Autodesk Inventor part; units mm, degrees
(part 7 of 11)
  arc A2531 (21.081, 10.0534) -> (21.1571, 10.058) centre (21.119, 10.0557) ccw
  line L1265 (21.082, 10.668) -> (21.119, 11.2803)
  arc A2532 (21.1571, 11.278) -> (21.081, 11.2826) centre (21.119, 11.2803) ccw
  arc A2533 (21.044, 10.6703) -> (21.12, 10.6657) centre (21.082, 10.668) ccw
  line L1266 (21.119, 11.2803) -> (21.2296, 11.8837)
  arc A2534 (21.2671, 11.8769) -> (21.1921, 11.8906) centre (21.2296, 11.8837) ccw
  arc A2535 (21.0816, 11.2872) -> (21.1565, 11.2735) centre (21.119, 11.2803) ccw
  line L1267 (21.2296, 11.8837) -> (21.4121, 12.4694)
  arc A2536 (21.4485, 12.4581) -> (21.3758, 12.4807) centre (21.4121, 12.4694) ccw
  arc A2537 (21.1933, 11.895) -> (21.266, 11.8724) centre (21.2296, 11.8837) ccw
  line L1268 (21.4121, 12.4694) -> (21.6639, 13.0288)
  arc A2538 (21.6986, 13.0132) -> (21.6291, 13.0444) centre (21.6639, 13.0288) ccw
  arc A2539 (21.3774, 12.485) -> (21.4469, 12.4537) centre (21.4121, 12.4694) ccw
  line L1269 (21.6639, 13.0288) -> (21.9812, 13.5538)
  arc A2540 (22.0138, 13.5341) -> (21.9486, 13.5735) centre (21.9812, 13.5538) ccw
  arc A2541 (21.6313, 13.0485) -> (21.6965, 13.0091) centre (21.6639, 13.0288) ccw
  line L1270 (21.9812, 13.5538) -> (22.3596, 14.0367)
  arc A2542 (22.3896, 14.0132) -> (22.3296, 14.0602) centre (22.3596, 14.0367) ccw
  arc A2543 (21.9512, 13.5773) -> (22.0112, 13.5303) centre (21.9812, 13.5538) ccw
  line L1271 (22.3596, 14.0367) -> (22.7933, 14.4704)
  arc A2544 (22.8203, 14.4435) -> (22.7664, 14.4974) centre (22.7933, 14.4704) ccw
  arc A2545 (22.3326, 14.0636) -> (22.3865, 14.0097) centre (22.3596, 14.0367) ccw
  line L1272 (22.7933, 14.4704) -> (23.2762, 14.8488)
  arc A2546 (23.2997, 14.8188) -> (23.2527, 14.8788) centre (23.2762, 14.8488) ccw
  arc A2547 (22.7698, 14.5004) -> (22.8168, 14.4404) centre (22.7933, 14.4704) ccw
  line L1273 (23.2762, 14.8488) -> (23.8012, 15.1661)
  arc A2548 (23.8209, 15.1335) -> (23.7815, 15.1987) centre (23.8012, 15.1661) ccw
  arc A2549 (23.2565, 14.8814) -> (23.2959, 14.8162) centre (23.2762, 14.8488) ccw
  line L1274 (23.8012, 15.1661) -> (24.3606, 15.4179)
  arc A2550 (24.3762, 15.3832) -> (24.3449, 15.4527) centre (24.3606, 15.4179) ccw
  arc A2551 (23.7855, 15.2009) -> (23.8168, 15.1314) centre (23.8012, 15.1661) ccw
  line L1275 (24.3606, 15.4179) -> (24.9463, 15.6003)
  arc A2552 (24.9576, 15.564) -> (24.9349, 15.6367) centre (24.9463, 15.6003) ccw
  arc A2553 (24.3492, 15.4543) -> (24.3719, 15.3815) centre (24.3606, 15.4179) ccw
  line L1276 (24.9463, 15.6003) -> (25.5497, 15.7109)
  arc A2554 (25.5566, 15.6734) -> (25.5428, 15.7483) centre (25.5497, 15.7108) ccw
  arc A2555 (24.9394, 15.6379) -> (24.9531, 15.5629) centre (24.9463, 15.6004) ccw
  line L1277 (25.5497, 15.7109) -> (26.162, 15.7478)
  arc A2556 (26.1643, 15.7098) -> (26.1597, 15.7858) centre (26.162, 15.7478) ccw
  arc A2557 (25.5474, 15.7489) -> (25.552, 15.6728) centre (25.5497, 15.7108) ccw
  line L1278 (26.162, 15.7478) -> (26.8194, 15.6894)
  arc A2558 (26.816, 15.6514) -> (26.8228, 15.7273) centre (26.8194, 15.6894) ccw
  arc A2559 (26.1654, 15.7858) -> (26.1586, 15.7099) centre (26.162, 15.7478) ccw
  line L1279 (26.8194, 15.6894) -> (27.464, 15.5482)
  arc A2560 (27.4559, 15.511) -> (27.4722, 15.5854) centre (27.464, 15.5482) ccw
  arc A2561 (26.8275, 15.7266) -> (26.8112, 15.6522) centre (26.8194, 15.6894) ccw
  line L1280 (27.464, 15.5482) -> (28.0857, 15.3267)
  arc A2562 (28.0729, 15.2908) -> (28.0985, 15.3626) centre (28.0857, 15.3267) ccw
  arc A2563 (27.4768, 15.5841) -> (27.4513, 15.5123) centre (27.464, 15.5482) ccw
  line L1281 (28.0857, 15.3267) -> (28.6745, 15.0285)
  arc A2564 (28.6573, 14.9945) -> (28.6917, 15.0625) centre (28.6745, 15.0285) ccw
  arc A2565 (28.1029, 15.3607) -> (28.0685, 15.2927) centre (28.0857, 15.3267) ccw
  line L1282 (28.6745, 15.0285) -> (29.2211, 14.6587)
  arc A2566 (29.1997, 14.6271) -> (29.2424, 14.6902) centre (29.2211, 14.6587) ccw
  arc A2567 (28.6959, 15.0601) -> (28.6532, 14.997) centre (28.6745, 15.0285) ccw
  line L1283 (29.2211, 14.6587) -> (29.7166, 14.2228)
  arc A2568 (29.691, 14.1936) -> (29.7413, 14.2507) centre (29.7162, 14.2222) ccw
  arc A2569 (29.2463, 14.6873) -> (29.1959, 14.6301) centre (29.2211, 14.6587) ccw
  line L1284 (29.7166, 14.2228) -> (29.8258, 13.5976)
  arc A2570 (29.7972, 13.5724) -> (29.8544, 13.6228) centre (29.8258, 13.5976) ccw
  arc A2571 (29.7447, 14.2473) -> (29.6876, 14.197) centre (29.7162, 14.2222) ccw
  line L1285 (29.8258, 13.5976) -> (29.8563, 12.9383)
  arc A2572 (30.491, 13.1592) -> (30.5541, 13.2019) centre (30.5225, 13.1805) ccw
  arc A2573 (29.8573, 13.6189) -> (29.7942, 13.5762) centre (29.8258, 13.5976) ccw
  line L1286 (29.8563, 12.9383) -> (29.8033, 12.2805)
  arc A2574 (29.7654, 12.2835) -> (29.8373, 12.2977) centre (29.8033, 12.2805) ccw
  arc A2575 (30.5565, 13.1977) -> (30.4885, 13.1633) centre (30.5225, 13.1805) ccw
  line L1287 (29.8033, 12.2805) -> (31.0422, 11.97)
  arc A2576 (31.0063, 11.9573) -> (31.0781, 11.9828) centre (31.0422, 11.97) ccw
  arc A2577 (29.8406, 12.2727) -> (29.7674, 12.2677) centre (29.8033, 12.2805) ccw
  line L1288 (31.0422, 11.97) -> (31.1834, 11.3254)
  arc A2578 (31.1462, 11.3172) -> (31.2206, 11.3335) centre (31.1834, 11.3254) ccw
  arc A2579 (31.0794, 11.9782) -> (31.005, 11.9619) centre (31.0422, 11.97) ccw
  line L1289 (31.1834, 11.3254) -> (31.3469, 10.7676)
  arc A2580 (31.3089, 10.7642) -> (31.3848, 10.771) centre (31.3469, 10.7676) ccw
  arc A2581 (31.2213, 11.3288) -> (31.1454, 11.322) centre (31.1834, 11.3254) ccw
  line L1290 (31.3469, 10.7676) -> (30.0789, 10.6966)
  arc A2582 (30.0753, 10.7345) -> (30.0789, 10.6585) centre (30.0789, 10.6966) ccw
  arc A2583 (31.3469, 10.7295) -> (31.3469, 10.8057) centre (31.3469, 10.7676) ccw
  line L1291 (30.0789, 10.6966) -> (30.0301, 11.2202)
  arc A2584 (30.0681, 11.2237) -> (29.9922, 11.2166) centre (30.0301, 11.2201) ccw
  arc A2585 (30.0408, 10.6952) -> (30.1169, 10.698) centre (30.0789, 10.6966) ccw
  line L1292 (30.0301, 11.2202) -> (29.9074, 11.7314)
  arc A2586 (29.9449, 11.7382) -> (29.8699, 11.7246) centre (29.9074, 11.7314) ccw
  arc A2587 (29.9926, 11.2133) -> (30.0676, 11.227) centre (30.0301, 11.2201) ccw
  line L1293 (29.9074, 11.7314) -> (29.7131, 12.22)
  arc A2588 (29.7281, 12.2215) -> (29.6558, 12.1974) centre (29.6919, 12.2094) ccw
  arc A2589 (29.8712, 11.7193) -> (29.9435, 11.7435) centre (29.9074, 11.7314) ccw
  line L1294 (29.7131, 12.22) -> (29.4514, 12.6758)
  arc A2590 (29.4855, 12.6929) -> (29.4174, 12.6587) centre (29.4514, 12.6758) ccw
  arc A2591 (29.6579, 12.1924) -> (29.726, 12.2265) centre (29.6919, 12.2094) ccw
  line L1295 (29.4514, 12.6758) -> (29.158, 13.1122)
  arc A2592 (29.1892, 13.134) -> (29.1267, 13.0905) centre (29.158, 13.1122) ccw
  arc A2593 (29.4201, 12.654) -> (29.4827, 12.6976) centre (29.4514, 12.6758) ccw
  line L1296 (29.158, 13.1122) -> (28.7968, 13.4952)
  arc A2594 (28.8247, 13.5212) -> (28.769, 13.4693) centre (28.7968, 13.4952) ccw
  arc A2595 (29.1301, 13.0862) -> (29.1858, 13.1382) centre (29.158, 13.1122) ccw
  line L1297 (28.7968, 13.4952) -> (28.387, 13.8247)
  arc A2596 (28.4109, 13.8544) -> (28.3631, 13.795) centre (28.387, 13.8247) ccw
  arc A2597 (28.773, 13.4655) -> (28.8207, 13.5249) centre (28.7968, 13.4952) ccw
  line L1298 (28.387, 13.8247) -> (27.9346, 14.0922)
  arc A2598 (27.9539, 14.125) -> (27.9152, 14.0595) centre (27.9345, 14.0923) ccw
  arc A2599 (28.3676, 13.7919) -> (28.4064, 13.8575) centre (28.387, 13.8247) ccw
  line L1299 (27.9346, 14.0922) -> (27.4486, 14.2929)
  arc A2600 (27.463, 14.3282) -> (27.4339, 14.2578) centre (27.4485, 14.293) ccw
  arc A2601 (27.92, 14.057) -> (27.9491, 14.1275) centre (27.9345, 14.0923) ccw
  line L1300 (27.4486, 14.2929) -> (26.939, 14.4224)
  arc A2602 (26.9482, 14.4594) -> (26.9295, 14.3855) centre (26.9388, 14.4224) ccw
  arc A2603 (27.4393, 14.256) -> (27.458, 14.3298) centre (27.4486, 14.2929) ccw
  line L1301 (26.939, 14.4224) -> (26.416, 14.478)
  arc A2604 (26.42, 14.5159) -> (26.412, 14.4401) centre (26.416, 14.478) ccw
  arc A2605 (26.9348, 14.3846) -> (26.9429, 14.4603) centre (26.9388, 14.4224) ccw
  line L1302 (26.416, 14.478) -> (26.162, 14.478)
  arc A2606 (26.162, 14.5161) -> (26.162, 14.4399) centre (26.162, 14.478) ccw
  arc A2607 (26.416, 14.4399) -> (26.416, 14.5161) centre (26.416, 14.478) ccw
  line L1303 (26.162, 14.478) -> (25.6198, 14.4392)
  arc A2608 (25.6171, 14.4772) -> (25.6225, 14.4012) centre (25.6198, 14.4392) ccw
  arc A2609 (26.1647, 14.44) -> (26.1593, 14.516) centre (26.162, 14.478) ccw
  line L1304 (25.6198, 14.4392) -> (25.0886, 14.3237)
  arc A2610 (25.0805, 14.3609) -> (25.0967, 14.2864) centre (25.0886, 14.3237) ccw
  arc A2611 (25.6279, 14.402) -> (25.6117, 14.4764) centre (25.6198, 14.4392) ccw
  line L1305 (25.0886, 14.3237) -> (24.5793, 14.1337)
  arc A2612 (24.566, 14.1694) -> (24.5926, 14.098) centre (24.5793, 14.1337) ccw
  arc A2613 (25.1019, 14.288) -> (25.0753, 14.3594) centre (25.0886, 14.3237) ccw
  line L1306 (24.5793, 14.1337) -> (24.1022, 13.8732)
  arc A2614 (24.0839, 13.9066) -> (24.1204, 13.8397) centre (24.1022, 13.8732) ccw
  arc A2615 (24.5975, 14.1003) -> (24.561, 14.1671) centre (24.5793, 14.1337) ccw
  line L1307 (24.1022, 13.8732) -> (23.667, 13.5474)
  arc A2616 (23.6441, 13.5779) -> (23.6898, 13.5169) centre (23.667, 13.5474) ccw
  arc A2617 (24.125, 13.8427) -> (24.0793, 13.9037) centre (24.1022, 13.8732) ccw
  line L1308 (23.667, 13.5474) -> (23.2826, 13.163)
  arc A2618 (23.2557, 13.19) -> (23.3095, 13.1361) centre (23.2826, 13.163) ccw
  arc A2619 (23.6939, 13.5205) -> (23.64, 13.5743) centre (23.667, 13.5474) ccw
  line L1309 (23.2826, 13.163) -> (22.9568, 12.7278)
  arc A2620 (22.9263, 12.7507) -> (22.9873, 12.705) centre (22.9568, 12.7278) ccw
  arc A2621 (23.3131, 13.1402) -> (23.2521, 13.1859) centre (23.2826, 13.163) ccw
  line L1310 (22.9568, 12.7278) -> (22.6963, 12.2507)
  arc A2622 (22.6629, 12.269) -> (22.7297, 12.2325) centre (22.6963, 12.2507) ccw
  arc A2623 (22.9903, 12.7096) -> (22.9234, 12.7461) centre (22.9568, 12.7278) ccw
  line L1311 (22.6963, 12.2507) -> (22.5063, 11.7414)
  arc A2624 (22.4706, 11.7547) -> (22.542, 11.7281) centre (22.5063, 11.7414) ccw
  arc A2625 (22.732, 12.2374) -> (22.6606, 12.264) centre (22.6963, 12.2507) ccw
  line L1312 (22.5063, 11.7414) -> (22.3908, 11.2102)
  arc A2626 (22.3535, 11.2183) -> (22.428, 11.2021) centre (22.3908, 11.2102) ccw
  arc A2627 (22.5436, 11.7333) -> (22.4691, 11.7495) centre (22.5063, 11.7414) ccw
  line L1313 (22.3908, 11.2102) -> (22.352, 10.668)
  arc A2628 (22.314, 10.6707) -> (22.39, 10.6653) centre (22.352, 10.668) ccw
  arc A2629 (22.4288, 11.2075) -> (22.3528, 11.2129) centre (22.3908, 11.2102) ccw
  line L1314 (22.352, 10.668) -> (22.3908, 10.1258)
  arc A2630 (22.3528, 10.1231) -> (22.4288, 10.1285) centre (22.3908, 10.1258) ccw
  arc A2631 (22.39, 10.6707) -> (22.314, 10.6653) centre (22.352, 10.668) ccw
  line L1315 (22.3908, 10.1258) -> (22.5063, 9.5946)
  arc A2632 (22.4691, 9.5865) -> (22.5436, 9.6027) centre (22.5063, 9.5946) ccw
  arc A2633 (22.428, 10.1339) -> (22.3535, 10.1177) centre (22.3908, 10.1258) ccw
  line L1316 (22.5063, 9.5946) -> (22.6963, 9.0853)
  arc A2634 (22.6606, 9.072) -> (22.732, 9.0986) centre (22.6963, 9.0853) ccw
  arc A2635 (22.542, 9.6079) -> (22.4706, 9.5813) centre (22.5063, 9.5946) ccw
  line L1317 (22.6963, 9.0853) -> (22.9568, 8.6082)
  arc A2636 (22.9234, 8.5899) -> (22.9903, 8.6264) centre (22.9568, 8.6082) ccw
  arc A2637 (22.7297, 9.1035) -> (22.6629, 9.067) centre (22.6963, 9.0853) ccw
  line L1318 (22.9568, 8.6082) -> (23.2826, 8.173)
  arc A2638 (23.2521, 8.1501) -> (23.3131, 8.1958) centre (23.2826, 8.173) ccw
  arc A2639 (22.9873, 8.631) -> (22.9263, 8.5853) centre (22.9568, 8.6082) ccw
  line L1319 (23.2826, 8.173) -> (23.667, 7.7886)
  arc A2640 (23.64, 7.7617) -> (23.6939, 7.8155) centre (23.667, 7.7886) ccw
  arc A2641 (23.3095, 8.1999) -> (23.2557, 8.146) centre (23.2826, 8.173) ccw
  line L1320 (23.667, 7.7886) -> (24.1022, 7.4628)
  arc A2642 (24.0793, 7.4323) -> (24.125, 7.4933) centre (24.1022, 7.4628) ccw
  arc A2643 (23.6898, 7.8191) -> (23.6441, 7.7581) centre (23.667, 7.7886) ccw
  line L1321 (24.1022, 7.4628) -> (24.5793, 7.2023)
  arc A2644 (24.561, 7.1689) -> (24.5975, 7.2357) centre (24.5793, 7.2023) ccw
  arc A2645 (24.1204, 7.4963) -> (24.0839, 7.4294) centre (24.1022, 7.4628) ccw
  line L1322 (24.5793, 7.2023) -> (25.0886, 7.0123)
  arc A2646 (25.0753, 6.9766) -> (25.1019, 7.048) centre (25.0886, 7.0123) ccw
  arc A2647 (24.5926, 7.238) -> (24.566, 7.1666) centre (24.5793, 7.2023) ccw
  line L1323 (25.0886, 7.0123) -> (25.6198, 6.8968)
  arc A2648 (25.6117, 6.8595) -> (25.6279, 6.934) centre (25.6198, 6.8968) ccw
  arc A2649 (25.0967, 7.0496) -> (25.0805, 6.9751) centre (25.0886, 7.0123) ccw
  line L1324 (25.6198, 6.8968) -> (26.162, 6.858)
  arc A2650 (26.1593, 6.82) -> (26.1647, 6.896) centre (26.162, 6.858) ccw
  arc A2651 (25.6225, 6.9348) -> (25.6171, 6.8588) centre (25.6198, 6.8968) ccw
  line L1325 (26.162, 6.858) -> (26.6485, 6.8782)
  arc A2652 (26.65, 6.8402) -> (26.6469, 6.9163) centre (26.6485, 6.8782) ccw
  arc A2653 (26.1604, 6.8961) -> (26.1636, 6.8199) centre (26.162, 6.858) ccw
  line L1326 (26.6485, 6.8782) -> (27.1281, 6.9618)
  arc A2654 (27.1347, 6.9242) -> (27.1216, 6.9993) centre (27.1281, 6.9618) ccw
  arc A2655 (26.6419, 6.9158) -> (26.655, 6.8407) centre (26.6485, 6.8782) ccw
  line L1327 (27.1281, 6.9618) -> (27.5928, 7.1072)
  arc A2656 (27.6042, 7.0709) -> (27.5814, 7.1436) centre (27.5928, 7.1072) ccw
  arc A2657 (27.1167, 6.9982) -> (27.1395, 6.9254) centre (27.1281, 6.9618) ccw
  line L1328 (27.5928, 7.1072) -> (28.0345, 7.3121)
  arc A2658 (28.0505, 7.2775) -> (28.0184, 7.3466) centre (28.0345, 7.3121) ccw
  arc A2659 (27.5767, 7.1418) -> (27.6088, 7.0726) centre (27.5928, 7.1072) ccw
  line L1329 (28.0345, 7.3121) -> (28.4456, 7.5728)
  arc A2660 (28.466, 7.5406) -> (28.4252, 7.605) centre (28.4456, 7.5728) ccw
  arc A2661 (28.0141, 7.3443) -> (28.0549, 7.2799) centre (28.0345, 7.3121) ccw
  line L1330 (28.4456, 7.5728) -> (28.8192, 7.885)
  arc A2662 (28.8437, 7.8558) -> (28.7948, 7.9143) centre (28.8192, 7.885) ccw
  arc A2663 (28.4212, 7.602) -> (28.4701, 7.5436) centre (28.4456, 7.5728) ccw
  line L1331 (28.8192, 7.885) -> (29.1489, 8.2433)
  arc A2664 (29.177, 8.2175) -> (29.1209, 8.2691) centre (29.1489, 8.2433) ccw
  arc A2665 (28.7912, 7.9108) -> (28.8473, 7.8592) centre (28.8192, 7.885) ccw
  line L1332 (29.1489, 8.2433) -> (29.429, 8.6416)
  arc A2666 (29.4602, 8.6196) -> (29.3979, 8.6635) centre (29.429, 8.6416) ccw
  arc A2667 (29.1178, 8.2652) -> (29.1801, 8.2214) centre (29.1489, 8.2433) ccw
  line L1333 (29.429, 8.6416) -> (29.6547, 9.073)
  arc A2668 (29.6885, 9.0553) -> (29.621, 9.0906) centre (29.6547, 9.073) ccw
  arc A2669 (29.3953, 8.6592) -> (29.4628, 8.6239) centre (29.429, 8.6416) ccw
  line L1334 (29.6547, 9.073) -> (29.2095, 9.27)
  arc A2670 (29.858, 9.517) -> (29.7864, 9.5432) centre (29.8222, 9.5301) ccw
  arc A2671 (29.619, 9.0861) -> (29.6905, 9.0598) centre (29.6547, 9.073) ccw
  line L1335 (29.2095, 9.27) -> (28.7423, 9.4072)
  arc A2672 (28.7795, 9.3988) -> (28.7051, 9.4155) centre (28.7423, 9.4072) ccw
  arc A2673 (29.1723, 9.2783) -> (29.2467, 9.2616) centre (29.2095, 9.27) ccw
  line L1336 (28.7423, 9.4072) -> (28.2613, 9.4822)
  arc A2674 (28.2992, 9.4788) -> (28.2233, 9.4856) centre (28.2613, 9.4822) ccw
  arc A2675 (28.7044, 9.4106) -> (28.7803, 9.4038) centre (28.7423, 9.4072) ccw
  line L1337 (28.2613, 9.4822) -> (28.3443, 10.7495)
  arc A2676 (28.3443, 10.7114) -> (28.3443, 10.7876) centre (28.3443, 10.7495) ccw
  arc A2677 (28.2613, 9.5203) -> (28.2846, 9.4521) centre (28.2613, 9.4822) ccw
  line L1338 (21.1328, 9.9806) -> (21.1328, 11.3554)
  arc A2678 (21.1709, 11.3554) -> (21.0947, 11.3554) centre (21.1328, 11.3554) ccw
  arc A2679 (21.0947, 9.9806) -> (21.1709, 9.9806) centre (21.1328, 9.9806) ccw
  line L1339 (21.2852, 9.2739) -> (21.2852, 12.0621)
  arc A2680 (21.3233, 12.0621) -> (21.2471, 12.0621) centre (21.2852, 12.0621) ccw
  arc A2681 (21.2471, 9.2739) -> (21.3233, 9.2739) centre (21.2852, 9.2739) ccw
  line L1340 (21.4376, 8.81) -> (21.4376, 12.526)
  arc A2682 (21.4757, 12.526) -> (21.3995, 12.526) centre (21.4376, 12.526) ccw
  arc A2683 (21.3995, 8.81) -> (21.4757, 8.81) centre (21.4376, 8.81) ccw
  line L1341 (21.59, 8.4714) -> (21.59, 12.8646)
  arc A2684 (21.6281, 12.8646) -> (21.5519, 12.8646) centre (21.59, 12.8646) ccw
  arc A2685 (21.5519, 8.4714) -> (21.6281, 8.4714) centre (21.59, 8.4714) ccw
  line L1342 (21.7424, 8.1773) -> (21.7424, 13.1587)
  arc A2686 (21.7805, 13.1587) -> (21.7043, 13.1587) centre (21.7424, 13.1587) ccw
  arc A2687 (21.7043, 8.1773) -> (21.7805, 8.1773) centre (21.7424, 8.1773) ccw
  line L1343 (21.8948, 7.9252) -> (21.8948, 13.4108)
  arc A2688 (21.9329, 13.4108) -> (21.8567, 13.4108) centre (21.8948, 13.4108) ccw
  arc A2689 (21.8567, 7.9252) -> (21.9329, 7.9252) centre (21.8948, 7.9252) ccw
  line L1344 (22.0472, 7.698) -> (22.0472, 13.6379)
  arc A2690 (22.0853, 13.6379) -> (22.0091, 13.6379) centre (22.0472, 13.6379) ccw
  arc A2691 (22.0091, 7.698) -> (22.0853, 7.698) centre (22.0472, 7.698) ccw
  line L1345 (22.1996, 7.5035) -> (22.1996, 13.8325)
  arc A2692 (22.2377, 13.8325) -> (22.1615, 13.8325) centre (22.1996, 13.8325) ccw
  arc A2693 (22.1615, 7.5035) -> (22.2377, 7.5035) centre (22.1996, 7.5035) ccw
  line L1346 (22.352, 7.309) -> (22.352, 10.668)
  arc A2694 (22.3901, 10.668) -> (22.3139, 10.668) centre (22.352, 10.668) ccw
  arc A2695 (22.3139, 7.309) -> (22.3901, 7.309) centre (22.352, 7.309) ccw
  line L1347 (22.352, 10.668) -> (22.352, 14.027)
  arc A2696 (22.3901, 14.027) -> (22.3139, 14.027) centre (22.352, 14.027) ccw
  arc A2697 (22.3139, 10.668) -> (22.3901, 10.668) centre (22.352, 10.668) ccw
  line L1348 (22.5044, 7.1545) -> (22.5044, 9.6035)
  arc A2698 (22.5425, 9.6035) -> (22.4663, 9.6035) centre (22.5044, 9.6035) ccw
  arc A2699 (22.4663, 7.1545) -> (22.5425, 7.1545) centre (22.5044, 7.1545) ccw
  line L1349 (22.5044, 11.7325) -> (22.5044, 14.1815)
  arc A2700 (22.5425, 14.1815) -> (22.4663, 14.1815) centre (22.5044, 14.1815) ccw
  arc A2701 (22.4663, 11.7325) -> (22.5425, 11.7325) centre (22.5044, 11.7325) ccw
  line L1350 (22.6568, 7.0021) -> (22.6568, 9.1912)
  arc A2702 (22.6949, 9.1912) -> (22.6187, 9.1912) centre (22.6568, 9.1912) ccw
  arc A2703 (22.6187, 7.0021) -> (22.6949, 7.0021) centre (22.6568, 7.0021) ccw
  line L1351 (22.6568, 12.1448) -> (22.6568, 14.3339)
  arc A2704 (22.6949, 14.3339) -> (22.6187, 14.3339) centre (22.6568, 14.3339) ccw
  arc A2705 (22.6187, 12.1448) -> (22.6949, 12.1448) centre (22.6568, 12.1448) ccw
  line L1352 (22.8092, 6.8531) -> (22.8092, 8.8785)
  arc A2706 (22.8473, 8.8785) -> (22.7711, 8.8785) centre (22.8092, 8.8785) ccw
  arc A2707 (22.7711, 6.8531) -> (22.8473, 6.8531) centre (22.8092, 6.8531) ccw
  line L1353 (22.8092, 12.4575) -> (22.8092, 14.4828)
  arc A2708 (22.8473, 14.4828) -> (22.7711, 14.4828) centre (22.8092, 14.4828) ccw
  arc A2709 (22.7711, 12.4575) -> (22.8473, 12.4575) centre (22.8092, 12.4575) ccw
  line L1354 (22.9616, 6.7337) -> (22.9616, 8.6018)
  arc A2710 (22.9997, 8.6018) -> (22.9235, 8.6018) centre (22.9616, 8.6018) ccw
  arc A2711 (22.9235, 6.7337) -> (22.9997, 6.7337) centre (22.9616, 6.7337) ccw
  line L1355 (22.9616, 12.7342) -> (22.9616, 14.6023)
  arc A2712 (22.9997, 14.6023) -> (22.9235, 14.6023) centre (22.9616, 14.6023) ccw
  arc A2713 (22.9235, 12.7342) -> (22.9997, 12.7342) centre (22.9616, 12.7342) ccw
  line L1356 (23.114, 6.6143) -> (23.114, 8.3982)
  arc A2714 (23.1521, 8.3982) -> (23.0759, 8.3982) centre (23.114, 8.3982) ccw
  arc A2715 (23.0759, 6.6143) -> (23.1521, 6.6143) centre (23.114, 6.6143) ccw
  line L1357 (23.114, 12.9378) -> (23.114, 14.7217)
  arc A2716 (23.1521, 14.7217) -> (23.0759, 14.7217) centre (23.114, 14.7217) ccw
  arc A2717 (23.0759, 12.9378) -> (23.1521, 12.9378) centre (23.114, 12.9378) ccw
  line L1358 (23.2664, 6.4949) -> (23.2664, 8.1946)
  arc A2718 (23.3045, 8.1946) -> (23.2283, 8.1946) centre (23.2664, 8.1946) ccw
  arc A2719 (23.2283, 6.4949) -> (23.3045, 6.4949) centre (23.2664, 6.4949) ccw
  line L1359 (23.2664, 13.1414) -> (23.2664, 14.8411)
  arc A2720 (23.3045, 14.8411) -> (23.2283, 14.8411) centre (23.2664, 14.8411) ccw
  arc A2721 (23.2283, 13.1414) -> (23.3045, 13.1414) centre (23.2664, 13.1414) ccw
  line L1360 (23.4187, 6.401) -> (23.4188, 8.0367)
  arc A2722 (23.4569, 8.0367) -> (23.3807, 8.0367) centre (23.4188, 8.0367) ccw
  arc A2723 (23.3806, 6.401) -> (23.4568, 6.401) centre (23.4187, 6.401) ccw
  line L1361 (23.4188, 13.2993) -> (23.4188, 14.935)
  arc A2724 (23.4569, 14.935) -> (23.3807, 14.935) centre (23.4188, 14.935) ccw
  arc A2725 (23.3807, 13.2993) -> (23.4569, 13.2993) centre (23.4188, 13.2993) ccw
  line L1362 (23.5711, 6.3089) -> (23.5712, 7.8843)
  arc A2726 (23.6093, 7.8843) -> (23.5331, 7.8843) centre (23.5712, 7.8843) ccw
  arc A2727 (23.533, 6.3089) -> (23.6092, 6.3089) centre (23.5711, 6.3089) ccw
  line L1363 (23.5712, 13.4517) -> (23.5712, 15.0271)
  arc A2728 (23.6093, 15.0271) -> (23.5331, 15.0271) centre (23.5712, 15.0271) ccw
  arc A2729 (23.5331, 13.4517) -> (23.6093, 13.4517) centre (23.5712, 13.4517) ccw
  line L1364 (23.7235, 6.2167) -> (23.7236, 7.7462)
  arc A2730 (23.7617, 7.7462) -> (23.6855, 7.7462) centre (23.7236, 7.7462) ccw
  arc A2731 (23.6854, 6.2167) -> (23.7616, 6.2167) centre (23.7235, 6.2167) ccw
  line L1365 (23.7236, 13.5898) -> (23.7236, 15.1192)
  arc A2732 (23.7617, 15.1192) -> (23.6855, 15.1192) centre (23.7236, 15.1192) ccw
  arc A2733 (23.6855, 13.5898) -> (23.7617, 13.5898) centre (23.7236, 13.5898) ccw
  line L1366 (23.8759, 6.1361) -> (23.876, 7.632)
  arc A2734 (23.9141, 7.632) -> (23.8379, 7.632) centre (23.876, 7.632) ccw
  arc A2735 (23.8378, 6.1361) -> (23.914, 6.1361) centre (23.8759, 6.1361) ccw
  line L1367 (23.876, 13.7039) -> (23.876, 15.1998)
  arc A2736 (23.9141, 15.1998) -> (23.8379, 15.1998) centre (23.876, 15.1998) ccw
  arc A2737 (23.8379, 13.7039) -> (23.9141, 13.7039) centre (23.876, 13.7039) ccw
  line L1368 (24.0283, 6.0675) -> (24.0284, 7.518)
  arc A2738 (24.0665, 7.518) -> (23.9903, 7.518) centre (24.0284, 7.518) ccw
  arc A2739 (23.9902, 6.0675) -> (24.0664, 6.0675) centre (24.0283, 6.0675) ccw
  line L1369 (24.0284, 13.8179) -> (24.0284, 15.2684)
  arc A2740 (24.0665, 15.2684) -> (23.9903, 15.2684) centre (24.0284, 15.2684) ccw
  arc A2741 (23.9903, 13.8179) -> (24.0665, 13.8179) centre (24.0284, 13.8179) ccw
  line L1370 (24.1807, 5.9989) -> (24.1808, 7.4199)
  arc A2742 (24.2189, 7.4199) -> (24.1427, 7.4199) centre (24.1808, 7.4199) ccw
  arc A2743 (24.1426, 5.9989) -> (24.2188, 5.9989) centre (24.1807, 5.9989) ccw
  line L1371 (24.1808, 13.9161) -> (24.1808, 15.337)
  arc A2744 (24.2189, 15.337) -> (24.1427, 15.337) centre (24.1808, 15.337) ccw
  arc A2745 (24.1427, 13.9161) -> (24.2189, 13.9161) centre (24.1808, 13.9161) ccw
  line L1372 (24.3332, 5.9304) -> (24.3332, 7.3367)
  arc A2746 (24.3713, 7.3367) -> (24.2951, 7.3367) centre (24.3332, 7.3367) ccw
  arc A2747 (24.2951, 5.9304) -> (24.3713, 5.9304) centre (24.3332, 5.9304) ccw
  line L1373 (24.3332, 13.9993) -> (24.3332, 15.4056)
  arc A2748 (24.3713, 15.4056) -> (24.2951, 15.4056) centre (24.3332, 15.4056) ccw
  arc A2749 (24.2951, 13.9993) -> (24.3713, 13.9993) centre (24.3332, 13.9993) ccw
  line L1374 (24.4856, 5.8792) -> (24.4856, 7.2534)
  arc A2750 (24.5237, 7.2534) -> (24.4475, 7.2534) centre (24.4856, 7.2534) ccw
  arc A2751 (24.4475, 5.8792) -> (24.5237, 5.8792) centre (24.4856, 5.8792) ccw
  line L1375 (24.4856, 14.0825) -> (24.4856, 15.4568)
  arc A2752 (24.5237, 15.4568) -> (24.4475, 15.4568) centre (24.4856, 15.4568) ccw
  arc A2753 (24.4475, 14.0825) -> (24.5237, 14.0825) centre (24.4856, 14.0825) ccw
  line L1376 (24.638, 5.8317) -> (24.638, 7.1804)
  arc A2754 (24.6761, 7.1804) -> (24.5999, 7.1804) centre (24.638, 7.1804) ccw
  arc A2755 (24.5999, 5.8317) -> (24.6761, 5.8317) centre (24.638, 5.8317) ccw
  line L1377 (24.638, 14.1556) -> (24.638, 15.5043)
  arc A2756 (24.6761, 15.5043) -> (24.5999, 15.5043) centre (24.638, 15.5043) ccw
  arc A2757 (24.5999, 14.1556) -> (24.6761, 14.1556) centre (24.638, 14.1556) ccw
  line L1378 (24.7904, 5.7843) -> (24.7904, 7.1235)
  arc A2758 (24.8285, 7.1235) -> (24.7523, 7.1235) centre (24.7904, 7.1235) ccw
  arc A2759 (24.7523, 5.7843) -> (24.8285, 5.7843) centre (24.7904, 5.7843) ccw
  line L1379 (24.7904, 14.2124) -> (24.7904, 15.5518)
  arc A2760 (24.8285, 15.5518) -> (24.7523, 15.5518) centre (24.7904, 15.5518) ccw
  arc A2761 (24.7523, 14.2124) -> (24.8285, 14.2124) centre (24.7904, 14.2124) ccw
  line L1380 (24.9428, 5.7367) -> (24.9428, 7.0667)
  arc A2762 (24.9809, 7.0667) -> (24.9047, 7.0667) centre (24.9428, 7.0667) ccw
  arc A2763 (24.9047, 5.7367) -> (24.9809, 5.7367) centre (24.9428, 5.7367) ccw
  line L1381 (24.9428, 14.2693) -> (24.9428, 15.5993)
  arc A2764 (24.9809, 15.5993) -> (24.9047, 15.5993) centre (24.9428, 15.5993) ccw
  arc A2765 (24.9047, 14.2693) -> (24.9809, 14.2693) centre (24.9428, 14.2693) ccw
  line L1382 (25.0952, 5.7083) -> (25.0952, 7.0109)
  arc A2766 (25.1333, 7.0109) -> (25.0571, 7.0109) centre (25.0952, 7.0109) ccw
  arc A2767 (25.0571, 5.7083) -> (25.1333, 5.7083) centre (25.0952, 5.7083) ccw
  line L1383 (25.0952, 14.3251) -> (25.0952, 15.6277)
  arc A2768 (25.1333, 15.6277) -> (25.0571, 15.6277) centre (25.0952, 15.6277) ccw
  arc A2769 (25.0571, 14.3251) -> (25.1333, 14.3251) centre (25.0952, 14.3251) ccw
  line L1384 (25.2476, 5.6807) -> (25.2476, 6.9777)
  arc A2770 (25.2857, 6.9777) -> (25.2095, 6.9777) centre (25.2476, 6.9777) ccw
  arc A2771 (25.2095, 5.6807) -> (25.2857, 5.6807) centre (25.2476, 5.6807) ccw
  line L1385 (25.2476, 14.3583) -> (25.2476, 15.6555)
  arc A2772 (25.2857, 15.6555) -> (25.2095, 15.6555) centre (25.2476, 15.6555) ccw
  arc A2773 (25.2095, 14.3583) -> (25.2857, 14.3583) centre (25.2476, 14.3583) ccw
  line L1386 (25.4, 5.6528) -> (25.4, 6.9446)
  arc A2774 (25.4381, 6.9446) -> (25.3619, 6.9446) centre (25.4, 6.9446) ccw
  arc A2775 (25.3619, 5.6528) -> (25.4381, 5.6528) centre (25.4, 5.6528) ccw
  line L1387 (25.4, 14.3914) -> (25.4, 15.6834)
  arc A2776 (25.4381, 15.6834) -> (25.3619, 15.6834) centre (25.4, 15.6834) ccw
  arc A2777 (25.3619, 14.3914) -> (25.4381, 14.3914) centre (25.4, 14.3914) ccw
  line L1388 (25.5524, 5.6249) -> (25.5524, 6.9114)
  arc A2778 (25.5905, 6.9114) -> (25.5143, 6.9114) centre (25.5524, 6.9114) ccw
  arc A2779 (25.5143, 5.6249) -> (25.5905, 5.6249) centre (25.5524, 5.6249) ccw
  line L1389 (25.5524, 14.4246) -> (25.5524, 15.7111)
  arc A2780 (25.5905, 15.7111) -> (25.5143, 15.7111) centre (25.5524, 15.7111) ccw
  arc A2781 (25.5143, 14.4246) -> (25.5905, 14.4246) centre (25.5524, 14.4246) ccw
  line L1390 (25.7049, 5.6161) -> (25.7043, 6.8912)
  arc A2782 (25.7424, 6.8912) -> (25.6662, 6.8912) centre (25.7043, 6.8912) ccw
  arc A2783 (25.6668, 5.6161) -> (25.743, 5.6161) centre (25.7049, 5.6161) ccw
  line L1391 (25.7047, 14.4452) -> (25.7048, 15.7202)
  arc A2784 (25.7429, 15.7202) -> (25.6667, 15.7202) centre (25.7048, 15.7202) ccw
  arc A2785 (25.6666, 14.4452) -> (25.7428, 14.4452) centre (25.7047, 14.4452) ccw
  line L1392 (25.8573, 5.607) -> (25.8572, 6.8798)
  arc A2786 (25.8953, 6.8798) -> (25.8191, 6.8798) centre (25.8572, 6.8798) ccw
  arc A2787 (25.8192, 5.607) -> (25.8954, 5.607) centre (25.8573, 5.607) ccw
  line L1393 (25.8572, 14.4562) -> (25.8572, 15.7294)
  arc A2788 (25.8953, 15.7294) -> (25.8191, 15.7294) centre (25.8572, 15.7294) ccw
  arc A2789 (25.8191, 14.4562) -> (25.8953, 14.4562) centre (25.8572, 14.4562) ccw
  line L1394 (26.0097, 5.5978) -> (26.0096, 6.8689)
  arc A2790 (26.0477, 6.8689) -> (25.9715, 6.8689) centre (26.0096, 6.8689) ccw
  arc A2791 (25.9716, 5.5978) -> (26.0478, 5.5978) centre (26.0097, 5.5978) ccw
  line L1395 (26.0096, 14.4671) -> (26.0096, 15.7386)
  arc A2792 (26.0477, 15.7386) -> (25.9715, 15.7386) centre (26.0096, 15.7386) ccw
  arc A2793 (25.9715, 14.4671) -> (26.0477, 14.4671) centre (26.0096, 14.4671) ccw
  line L1396 (26.1621, 5.5887) -> (26.162, 6.858)
  arc A2794 (26.2001, 6.858) -> (26.1239, 6.858) centre (26.162, 6.858) ccw
  arc A2795 (26.124, 5.5887) -> (26.2002, 5.5887) centre (26.1621, 5.5887) ccw
  line L1397 (26.162, 14.478) -> (26.162, 15.7478)
  arc A2796 (26.2001, 15.7478) -> (26.1239, 15.7478) centre (26.162, 15.7478) ccw
  arc A2797 (26.1239, 14.478) -> (26.2001, 14.478) centre (26.162, 14.478) ccw
  line L1398 (26.3144, 5.5953) -> (26.3144, 6.8643)
  arc A2798 (26.3525, 6.8643) -> (26.2763, 6.8643) centre (26.3144, 6.8643) ccw
  arc A2799 (26.2763, 5.5953) -> (26.3525, 5.5953) centre (26.3144, 5.5953) ccw
  line L1399 (26.3148, 14.478) -> (26.3144, 15.7343)
  arc A2800 (26.3525, 15.7343) -> (26.2763, 15.7343) centre (26.3144, 15.7343) ccw
  arc A2801 (26.2767, 14.478) -> (26.3529, 14.478) centre (26.3148, 14.478) ccw
  line L1400 (26.4669, 5.6019) -> (26.4668, 6.8707)
  arc A2802 (26.5049, 6.8707) -> (26.4287, 6.8707) centre (26.4668, 6.8707) ccw
  arc A2803 (26.4288, 5.6019) -> (26.505, 5.6019) centre (26.4669, 5.6019) ccw
  line L1401 (26.4672, 14.4725) -> (26.4668, 15.7207)
  arc A2804 (26.5049, 15.7207) -> (26.4287, 15.7207) centre (26.4668, 15.7207) ccw
  arc A2805 (26.4291, 14.4725) -> (26.5053, 14.4725) centre (26.4672, 14.4725) ccw
  line L1402 (26.6193, 5.6085) -> (26.6192, 6.877)
  arc A2806 (26.6573, 6.877) -> (26.5811, 6.877) centre (26.6192, 6.877) ccw
  arc A2807 (26.5812, 5.6085) -> (26.6574, 5.6085) centre (26.6193, 5.6085) ccw
  line L1403 (26.6196, 14.4563) -> (26.6192, 15.7072)
  arc A2808 (26.6573, 15.7072) -> (26.5811, 15.7072) centre (26.6192, 15.7072) ccw
  arc A2809 (26.5815, 14.4563) -> (26.6577, 14.4563) centre (26.6196, 14.4563) ccw
  line L1404 (26.7717, 5.615) -> (26.7716, 6.8997)
  arc A2810 (26.8097, 6.8997) -> (26.7335, 6.8997) centre (26.7716, 6.8997) ccw
  arc A2811 (26.7336, 5.615) -> (26.8098, 5.615) centre (26.7717, 5.615) ccw
  line L1405 (26.772, 14.4402) -> (26.7716, 15.6936)
  arc A2812 (26.8097, 15.6936) -> (26.7335, 15.6936) centre (26.7716, 15.6936) ccw
  arc A2813 (26.7339, 14.4402) -> (26.8101, 14.4402) centre (26.772, 14.4402) ccw
  line L1406 (26.924, 5.6389) -> (26.924, 6.9262)
  arc A2814 (26.9621, 6.9262) -> (26.8859, 6.9262) centre (26.924, 6.9262) ccw
  arc A2815 (26.8859, 5.6389) -> (26.9621, 5.6389) centre (26.924, 5.6389) ccw
  line L1407 (26.9242, 14.4239) -> (26.924, 15.6665)
  arc A2816 (26.9621, 15.6665) -> (26.8859, 15.6665) centre (26.924, 15.6665) ccw
  arc A2817 (26.8861, 14.4239) -> (26.9623, 14.4239) centre (26.9242, 14.4239) ccw
  line L1408 (27.0758, 5.6694) -> (27.0764, 6.9528)
  arc A2818 (27.1145, 6.9528) -> (27.0383, 6.9528) centre (27.0764, 6.9528) ccw
  arc A2819 (27.0377, 5.6694) -> (27.1139, 5.6694) centre (27.0758, 5.6694) ccw
  line L1409 (27.0764, 14.3875) -> (27.0764, 15.6331)
  arc A2820 (27.1145, 15.6331) -> (27.0383, 15.6331) centre (27.0764, 15.6331) ccw
  arc A2821 (27.0383, 14.3875) -> (27.1145, 14.3875) centre (27.0764, 14.3875) ccw
  line L1410 (27.2276, 5.6999) -> (27.2288, 6.9933)
  arc A2822 (27.2669, 6.9933) -> (27.1907, 6.9933) centre (27.2288, 6.9933) ccw
  arc A2823 (27.1895, 5.6999) -> (27.2657, 5.6999) centre (27.2276, 5.6999) ccw
  line L1411 (27.229, 14.3487) -> (27.2288, 15.5997)
  arc A2824 (27.2669, 15.5997) -> (27.1907, 15.5997) centre (27.2288, 15.5997) ccw
  arc A2825 (27.1909, 14.3487) -> (27.2671, 14.3487) centre (27.229, 14.3487) ccw
  line L1412 (27.3794, 5.7304) -> (27.3812, 7.041)
  arc A2826 (27.4193, 7.041) -> (27.3431, 7.041) centre (27.3812, 7.041) ccw
  arc A2827 (27.3413, 5.7304) -> (27.4175, 5.7304) centre (27.3794, 5.7304) ccw
  line L1413 (27.3812, 14.3101) -> (27.3812, 15.5663)
  arc A2828 (27.4193, 15.5663) -> (27.3431, 15.5663) centre (27.3812, 15.5663) ccw
  arc A2829 (27.3431, 14.3101) -> (27.4193, 14.3101) centre (27.3812, 14.3101) ccw
  line L1414 (27.5326, 5.769) -> (27.5336, 7.0887)
  arc A2830 (27.5717, 7.0887) -> (27.4955, 7.0887) centre (27.5336, 7.0887) ccw
  arc A2831 (27.4945, 5.769) -> (27.5707, 5.769) centre (27.5326, 5.769) ccw
  line L1415 (27.5335, 14.2579) -> (27.5336, 15.5234)
  arc A2832 (27.5717, 15.5234) -> (27.4955, 15.5234) centre (27.5336, 15.5234) ccw
  arc A2833 (27.4954, 14.2579) -> (27.5716, 14.2579) centre (27.5335, 14.2579) ccw
  line L1416 (27.686, 5.8083) -> (27.686, 7.1505)
  arc A2834 (27.7241, 7.1505) -> (27.6479, 7.1505) centre (27.686, 7.1505) ccw
  arc A2835 (27.6479, 5.8083) -> (27.7241, 5.8083) centre (27.686, 5.8083) ccw
  line L1417 (27.6862, 14.1948) -> (27.686, 15.4691)
  arc A2836 (27.7241, 15.4691) -> (27.6479, 15.4691) centre (27.686, 15.4691) ccw
  arc A2837 (27.6481, 14.1948) -> (27.7243, 14.1948) centre (27.6862, 14.1948) ccw
  line L1418 (27.8384, 5.8571) -> (27.8384, 7.2211)
  arc A2838 (27.8765, 7.2211) -> (27.8003, 7.2211) centre (27.8384, 7.2211) ccw
  arc A2839 (27.8003, 5.8571) -> (27.8765, 5.8571) centre (27.8384, 5.8571) ccw
  line L1419 (27.8383, 14.132) -> (27.8384, 15.4148)
  arc A2840 (27.8765, 15.4148) -> (27.8003, 15.4148) centre (27.8384, 15.4148) ccw
  arc A2841 (27.8002, 14.132) -> (27.8764, 14.132) centre (27.8383, 14.132) ccw
  line L1420 (27.9922, 5.9077) -> (27.9908, 7.2918)
  arc A2842 (28.0289, 7.2918) -> (27.9527, 7.2918) centre (27.9908, 7.2918) ccw
  arc A2843 (27.9541, 5.9077) -> (28.0303, 5.9077) centre (27.9922, 5.9077) ccw
  line L1421 (27.9909, 14.059) -> (27.9906, 15.3604)
  arc A2844 (28.0287, 15.3604) -> (27.9525, 15.3604) centre (27.9906, 15.3604) ccw
  arc A2845 (27.9528, 14.059) -> (28.029, 14.059) centre (27.9909, 14.059) ccw
  line L1422 (28.1432, 5.9642) -> (28.1432, 7.381)
  arc A2846 (28.1813, 7.381) -> (28.1051, 7.381) centre (28.1432, 7.381) ccw
  arc A2847 (28.1051, 5.9642) -> (28.1813, 5.9642) centre (28.1432, 5.9642) ccw
  line L1423 (28.1433, 13.9688) -> (28.1431, 15.2976)
  arc A2848 (28.1812, 15.2976) -> (28.105, 15.2976) centre (28.1431, 15.2976) ccw
  arc A2849 (28.1052, 13.9688) -> (28.1814, 13.9688) centre (28.1433, 13.9688) ccw
  line L1424 (28.2955, 6.0361) -> (28.2956, 7.4777)
  arc A2850 (28.3337, 7.4777) -> (28.2575, 7.4777) centre (28.2956, 7.4777) ccw
  arc A2851 (28.2574, 6.0361) -> (28.3336, 6.0361) centre (28.2955, 6.0361) ccw
  line L1425 (28.2957, 13.8787) -> (28.2954, 15.2204)
  arc A2852 (28.3335, 15.2204) -> (28.2573, 15.2204) centre (28.2954, 15.2204) ccw
  arc A2853 (28.2576, 13.8787) -> (28.3338, 13.8787) centre (28.2957, 13.8787) ccw
  line L1426 (28.4481, 6.1079) -> (28.448, 7.5748)
  arc A2854 (28.4861, 7.5748) -> (28.4099, 7.5748) centre (28.448, 7.5748) ccw
  arc A2855 (28.41, 6.1079) -> (28.4862, 6.1079) centre (28.4481, 6.1079) ccw
  line L1427 (28.448, 13.7757) -> (28.4479, 15.1432)
  arc A2856 (28.486, 15.1432) -> (28.4098, 15.1432) centre (28.4479, 15.1432) ccw
  arc A2857 (28.4099, 13.7757) -> (28.4861, 13.7757) centre (28.448, 13.7757) ccw
  line L1428 (28.6004, 6.1797) -> (28.6004, 7.7021)
  arc A2858 (28.6385, 7.7021) -> (28.5623, 7.7021) centre (28.6004, 7.7021) ccw
  arc A2859 (28.5623, 6.1797) -> (28.6385, 6.1797) centre (28.6004, 6.1797) ccw
  line L1429 (28.6004, 13.6531) -> (28.6003, 15.066)
  arc A2860 (28.6384, 15.066) -> (28.5622, 15.066) centre (28.6003, 15.066) ccw
  arc A2861 (28.5623, 13.6531) -> (28.6385, 13.6531) centre (28.6004, 13.6531) ccw
  line L1430 (28.7528, 6.2658) -> (28.7528, 7.8295)
  arc A2862 (28.7909, 7.8295) -> (28.7147, 7.8295) centre (28.7528, 7.8295) ccw
  arc A2863 (28.7147, 6.2658) -> (28.7909, 6.2658) centre (28.7528, 6.2658) ccw
  line L1431 (28.7528, 13.5306) -> (28.7528, 14.9755)
  arc A2864 (28.7909, 14.9755) -> (28.7147, 14.9755) centre (28.7528, 14.9755) ccw
  arc A2865 (28.7147, 13.5306) -> (28.7909, 13.5306) centre (28.7528, 13.5306) ccw
  line L1432 (28.9052, 6.3637) -> (28.9052, 7.9784)
  arc A2866 (28.9433, 7.9784) -> (28.8671, 7.9784) centre (28.9052, 7.9784) ccw
  arc A2867 (28.8671, 6.3637) -> (28.9433, 6.3637) centre (28.9052, 6.3637) ccw
  line L1433 (28.9062, 13.3792) -> (28.9052, 14.8724)
  arc A2868 (28.9433, 14.8724) -> (28.8671, 14.8724) centre (28.9052, 14.8724) ccw
  arc A2869 (28.8681, 13.3792) -> (28.9443, 13.3792) centre (28.9062, 13.3792) ccw
  line L1434 (29.0575, 6.4617) -> (29.0576, 8.144)
  arc A2870 (29.0957, 8.144) -> (29.0195, 8.144) centre (29.0576, 8.144) ccw
  arc A2871 (29.0194, 6.4617) -> (29.0956, 6.4617) centre (29.0575, 6.4617) ccw
  line L1435 (29.0594, 13.2167) -> (29.0577, 14.7692)
  arc A2872 (29.0958, 14.7692) -> (29.0196, 14.7692) centre (29.0577, 14.7692) ccw
  arc A2873 (29.0213, 13.2167) -> (29.0975, 13.2167) centre (29.0594, 13.2167) ccw
  line L1436 (29.21, 6.5596) -> (29.21, 8.3301)
  arc A2874 (29.2481, 8.3301) -> (29.1719, 8.3301) centre (29.21, 8.3301) ccw
  arc A2875 (29.1719, 6.5596) -> (29.2481, 6.5596) centre (29.21, 6.5596) ccw
  line L1437 (29.2112, 13.033) -> (29.2102, 14.666)
  arc A2876 (29.2483, 14.666) -> (29.1721, 14.666) centre (29.2102, 14.666) ccw
  arc A2877 (29.1731, 13.033) -> (29.2493, 13.033) centre (29.2112, 13.033) ccw
  line L1438 (29.3624, 6.6868) -> (29.3624, 8.5468)
  arc A2878 (29.4005, 8.5468) -> (29.3243, 8.5468) centre (29.3624, 8.5468) ccw
  arc A2879 (29.3243, 6.6868) -> (29.4005, 6.6868) centre (29.3624, 6.6868) ccw
  line L1439 (29.36, 12.8117) -> (29.3879, 14.5314)
  arc A2880 (29.426, 14.5314) -> (29.3498, 14.5314) centre (29.3879, 14.5314) ccw
  arc A2881 (29.3219, 12.8117) -> (29.3981, 12.8117) centre (29.36, 12.8117) ccw
  line L1440 (29.5148, 6.8157) -> (29.5148, 8.8055)
  arc A2882 (29.5529, 8.8055) -> (29.4767, 8.8055) centre (29.5148, 8.8055) ccw
  arc A2883 (29.4767, 6.8157) -> (29.5529, 6.8157) centre (29.5148, 6.8157) ccw
  line L1441 (29.5163, 12.5627) -> (29.5152, 14.4)
  arc A2884 (29.5533, 14.4) -> (29.4771, 14.4) centre (29.5152, 14.4) ccw
  arc A2885 (29.4782, 12.5627) -> (29.5544, 12.5627) centre (29.5163, 12.5627) ccw
  line L1442 (29.6672, 6.9446) -> (29.6216, 9.0876)
  arc A2886 (29.6597, 9.0876) -> (29.5835, 9.0876) centre (29.6216, 9.0876) ccw
  arc A2887 (29.6291, 6.9446) -> (29.7053, 6.9446) centre (29.6672, 6.9446) ccw
  line L1443 (29.6857, 12.2678) -> (29.5736, 14.2712)
  arc A2888 (29.6117, 14.2712) -> (29.5355, 14.2712) centre (29.5736, 14.2712) ccw
  arc A2889 (29.6476, 12.2678) -> (29.7238, 12.2678) centre (29.6857, 12.2678) ccw
  line L1444 (29.8196, 7.0995) -> (29.2164, 9.2669)
  arc A2890 (29.2545, 9.2669) -> (29.1783, 9.2669) centre (29.2164, 9.2669) ccw
  arc A2891 (29.7815, 7.0995) -> (29.8577, 7.0995) centre (29.8196, 7.0995) ccw
  line L1445 (29.8619, 11.8457) -> (29.7347, 14.1195)
  arc A2892 (29.7728, 14.1195) -> (29.6966, 14.1195) centre (29.7347, 14.1195) ccw
  arc A2893 (29.8238, 11.8457) -> (29.9, 11.8457) centre (29.8619, 11.8457) ccw
  line L1446 (29.972, 7.2672) -> (28.2613, 9.4822)
  arc A2894 (28.2638, 9.5202) -> (28.2232, 9.4822) centre (28.2613, 9.4822) ccw
  arc A2895 (29.9339, 7.2672) -> (30.0101, 7.2672) centre (29.972, 7.2672) ccw
  line L1447 (30.0789, 10.6966) -> (29.7789, 13.8664)
  arc A2896 (29.817, 13.8664) -> (29.7408, 13.8664) centre (29.7789, 13.8664) ccw
  arc A2897 (30.0408, 10.6966) -> (30.1169, 10.6987) centre (30.0789, 10.6966) ccw
  line L1448 (30.1244, 7.4349) -> (30.1244, 37.913)
  arc A2898 (30.1269, 37.9511) -> (30.1219, 37.875) centre (30.1244, 37.913) ccw
  arc A2899 (30.0863, 7.4349) -> (30.1625, 7.4349) centre (30.1244, 7.4349) ccw
  line L1449 (27.9445, 10.5772) -> (29.8185, 13.6393)
  arc A2900 (29.8566, 13.6393) -> (29.7804, 13.6393) centre (29.8185, 13.6393) ccw
  arc A2901 (27.9065, 10.575) -> (27.9825, 10.5793) centre (27.9445, 10.5772) ccw
  line L1450 (31.1218, 9.6002) -> (28.2812, 9.7864)
  arc A2902 (28.2837, 9.8244) -> (28.2787, 9.7484) centre (28.2812, 9.7864) ccw
  arc A2903 (31.0837, 9.6002) -> (31.1599, 9.6002) centre (31.1218, 9.6002) ccw
  line L1451 (28.1295, 10.5875) -> (29.8361, 13.376)
  arc A2904 (29.8742, 13.376) -> (29.798, 13.376) centre (29.8361, 13.376) ccw
  arc A2905 (28.0915, 10.5854) -> (28.1676, 10.5897) centre (28.1295, 10.5875) ccw
  line L1452 (30.4292, 7.863) -> (30.4292, 42.5643)
  arc A2906 (30.4317, 42.6023) -> (30.4267, 42.5263) centre (30.4292, 42.5643) ccw
  arc A2907 (30.3911, 7.863) -> (30.4673, 7.863) centre (30.4292, 7.863) ccw
  line L1453 (28.3145, 10.5979) -> (29.8486, 13.1046)
  arc A2908 (29.8867, 13.1046) -> (29.8105, 13.1046) centre (29.8486, 13.1046) ccw
  arc A2909 (28.2765, 10.5958) -> (28.3526, 10.6) centre (28.3145, 10.5979) ccw
  line L1454 (30.5816, 8.1088) -> (30.5816, 44.8899)
  arc A2910 (30.5841, 44.9279) -> (30.5791, 44.8519) centre (30.5816, 44.8899) ccw
  arc A2911 (30.5435, 8.1088) -> (30.6197, 8.1088) centre (30.5816, 8.1088) ccw
  line L1455 (28.4995, 10.6082) -> (29.8458, 12.808)
  arc A2912 (29.8839, 12.808) -> (29.8077, 12.808) centre (29.8458, 12.808) ccw
  arc A2913 (28.4615, 10.6061) -> (28.5376, 10.6104) centre (28.4995, 10.6082) ccw
  line L1456 (30.734, 8.4045) -> (30.7336, 47.2102)
  arc A2914 (30.7361, 47.2482) -> (30.7312, 47.1722) centre (30.7336, 47.2102) ccw
  arc A2915 (30.6959, 8.4045) -> (30.7721, 8.4045) centre (30.734, 8.4045) ccw
  line L1457 (28.6846, 10.6186) -> (29.8187, 12.4718)
  arc A2916 (29.8568, 12.4718) -> (29.7806, 12.4718) centre (29.8187, 12.4718) ccw
  arc A2917 (28.6465, 10.6165) -> (28.7226, 10.6207) centre (28.6846, 10.6186) ccw
  line L1458 (30.8864, 8.7493) -> (30.8864, 49.5411)
  arc A2918 (30.8889, 49.5791) -> (30.8839, 49.5031) centre (30.8864, 49.5411) ccw
  arc A2919 (30.8483, 8.7493) -> (30.9245, 8.7493) centre (30.8864, 8.7493) ccw
  line L1459 (32.1269, 10.8112) -> (29.9931, 12.2329)
  arc A2920 (30.0312, 12.2329) -> (29.955, 12.2329) centre (29.9931, 12.2329) ccw
  arc A2921 (32.0889, 10.8091) -> (32.165, 10.8134) centre (32.1269, 10.8112) ccw
  line L1460 (31.0388, 9.1733) -> (31.0388, 51.8666)
  arc A2922 (31.0413, 51.9046) -> (31.0363, 51.8286) centre (31.0388, 51.8666) ccw
  arc A2923 (31.0007, 9.1733) -> (31.0769, 9.1733) centre (31.0388, 9.1733) ccw
  line L1461 (32.3805, 10.8254) -> (30.4337, 12.1225)
  arc A2924 (30.4718, 12.1225) -> (30.3956, 12.1225) centre (30.4337, 12.1225) ccw
  arc A2925 (32.3424, 10.8233) -> (32.4185, 10.8275) centre (32.3805, 10.8254) ccw
  line L1462 (29.2003, 10.4756) -> (28.3394, 10.6739)
  arc A2926 (28.3419, 10.712) -> (28.3369, 10.6359) centre (28.3394, 10.6739) ccw
  arc A2927 (29.1622, 10.4756) -> (29.2384, 10.4756) centre (29.2003, 10.4756) ccw
  line L1463 (31.2989, 10.7649) -> (31.1963, 11.2814)
  arc A2928 (31.2344, 11.2814) -> (31.1582, 11.2814) centre (31.1963, 11.2814) ccw
  arc A2929 (31.2609, 10.7628) -> (31.337, 10.767) centre (31.2989, 10.7649) ccw
  line L1464 (10.4902, 5.588) -> (9.8395, 5.6423)
  arc A2930 (9.8426, 5.6803) -> (9.8363, 5.6043) centre (9.8395, 5.6423) ccw
  arc A2931 (10.487, 5.55) -> (10.4934, 5.626) centre (10.4902, 5.588) ccw
  line L1465 (9.8395, 5.6423) -> (9.2014, 5.7811)
  arc A2932 (9.2095, 5.8183) -> (9.1933, 5.7439) centre (9.2014, 5.7811) ccw
  arc A2933 (9.8314, 5.6051) -> (9.8476, 5.6795) centre (9.8395, 5.6423) ccw
  line L1466 (9.2014, 5.7811) -> (8.5869, 6.0019)
  arc A2934 (8.5998, 6.0378) -> (8.5741, 5.9661) centre (8.5869, 6.002) ccw
  arc A2935 (9.1885, 5.7452) -> (9.2143, 5.8169) centre (9.2014, 5.7811) ccw
  line L1467 (8.5869, 6.0019) -> (8.0066, 6.3011)
  arc A2936 (8.024, 6.335) -> (7.9891, 6.2673) centre (8.0066, 6.3011) ccw
  arc A2937 (8.5695, 5.9681) -> (8.6044, 6.0358) centre (8.5869, 6.0019) ccw
  line L1468 (8.0066, 6.3011) -> (7.4702, 6.6735)
  arc A2938 (7.4919, 6.7048) -> (7.4484, 6.6422) centre (7.4702, 6.6735) ccw
  arc A2939 (7.9848, 6.2698) -> (8.0283, 6.3324) centre (8.0065, 6.3011) ccw
  line L1469 (7.4702, 6.6735) -> (6.987, 7.1127)
  arc A2940 (7.0126, 7.1409) -> (6.9614, 7.0845) centre (6.987, 7.1127) ccw
  arc A2941 (7.4446, 6.6453) -> (7.4958, 6.7017) centre (7.4702, 6.6735) ccw
  line L1470 (6.987, 7.1127) -> (6.5653, 7.6112)
  arc A2942 (6.5944, 7.6358) -> (6.5362, 7.5866) centre (6.5653, 7.6112) ccw
  arc A2943 (6.9579, 7.0881) -> (7.0161, 7.1373) centre (6.987, 7.1127) ccw
  line L1471 (6.5653, 7.6112) -> (6.2122, 8.1605)
  arc A2944 (6.2443, 8.1811) -> (6.1802, 8.1399) centre (6.2122, 8.1605) ccw
  arc A2945 (6.5332, 7.5906) -> (6.5973, 7.6318) centre (6.5653, 7.6112) ccw
  line L1472 (6.2122, 8.1605) -> (5.9339, 8.7512)
  arc A2946 (5.9684, 8.7675) -> (5.8994, 8.735) centre (5.9339, 8.7512) ccw
  arc A2947 (6.1778, 8.1443) -> (6.2467, 8.1768) centre (6.2122, 8.1605) ccw
  line L1473 (5.9339, 8.7512) -> (5.7351, 9.3732)
  arc A2948 (5.7714, 9.3848) -> (5.6988, 9.3616) centre (5.7351, 9.3732) ccw
  arc A2949 (5.8976, 8.7396) -> (5.9702, 8.7628) centre (5.9339, 8.7512) ccw
  line L1474 (5.7351, 9.3732) -> (5.6191, 10.0158)
  arc A2950 (5.6566, 10.0225) -> (5.5816, 10.009) centre (5.6191, 10.0158) ccw
  arc A2951 (5.6976, 9.3664) -> (5.7726, 9.3799) centre (5.7351, 9.3732) ccw
  line L1475 (5.6191, 10.0158) -> (5.588, 10.668)
  arc A2952 (5.6261, 10.6698) -> (5.55, 10.6662) centre (5.588, 10.668) ccw
  arc A2953 (5.581, 10.0139) -> (5.6572, 10.0176) centre (5.6191, 10.0158) ccw
  line L1476 (5.588, 10.668) -> (5.625, 11.2803)
  arc A2954 (5.6631, 11.278) -> (5.587, 11.2826) centre (5.625, 11.2803) ccw
  arc A2955 (5.55, 10.6703) -> (5.626, 10.6657) centre (5.588, 10.668) ccw
  line L1477 (5.625, 11.2803) -> (5.7356, 11.8837)
  arc A2956 (5.7731, 11.8769) -> (5.6981, 11.8906) centre (5.7356, 11.8837) ccw
  arc A2957 (5.5876, 11.2872) -> (5.6625, 11.2734) centre (5.625, 11.2803) ccw
  line L1478 (5.7356, 11.8837) -> (5.9181, 12.4694)
  arc A2958 (5.9545, 12.4581) -> (5.8818, 12.4807) centre (5.9181, 12.4694) ccw
  arc A2959 (5.6993, 11.895) -> (5.772, 11.8724) centre (5.7356, 11.8837) ccw
  line L1479 (5.9181, 12.4694) -> (6.1699, 13.0288)
  arc A2960 (6.2046, 13.0131) -> (6.1351, 13.0444) centre (6.1699, 13.0288) ccw
  arc A2961 (5.8834, 12.485) -> (5.9529, 12.4537) centre (5.9181, 12.4694) ccw
  line L1480 (6.1699, 13.0288) -> (6.4872, 13.5538)
  arc A2962 (6.5199, 13.534) -> (6.4546, 13.5735) centre (6.4872, 13.5538) ccw
  arc A2963 (6.1373, 13.0485) -> (6.2025, 13.0091) centre (6.1699, 13.0288) ccw
  line L1481 (6.4872, 13.5538) -> (6.8656, 14.0367)
  arc A2964 (6.8956, 14.0131) -> (6.8356, 14.0602) centre (6.8656, 14.0367) ccw
  arc A2965 (6.4572, 13.5773) -> (6.5172, 13.5303) centre (6.4872, 13.5538) ccw
  line L1482 (6.8656, 14.0367) -> (7.2993, 14.4704)
  arc A2966 (7.3263, 14.4435) -> (7.2724, 14.4974) centre (7.2993, 14.4704) ccw
  arc A2967 (6.8386, 14.0636) -> (6.8925, 14.0097) centre (6.8656, 14.0367) ccw
  line L1483 (7.2993, 14.4704) -> (7.7822, 14.8488)
  arc A2968 (7.8057, 14.8188) -> (7.7587, 14.8788) centre (7.7822, 14.8488) ccw
  arc A2969 (7.2758, 14.5004) -> (7.3228, 14.4404) centre (7.2993, 14.4704) ccw
  line L1484 (7.7822, 14.8488) -> (8.3072, 15.1661)
  arc A2970 (8.3269, 15.1335) -> (8.2875, 15.1987) centre (8.3072, 15.1661) ccw
  arc A2971 (7.7625, 14.8814) -> (7.8019, 14.8161) centre (7.7822, 14.8488) ccw
  line L1485 (8.3072, 15.1661) -> (8.8666, 15.4179)
  arc A2972 (8.8823, 15.3831) -> (8.851, 15.4526) centre (8.8666, 15.4179) ccw
  arc A2973 (8.2916, 15.2009) -> (8.3228, 15.1314) centre (8.3072, 15.1661) ccw
  line L1486 (8.8666, 15.4179) -> (9.4523, 15.6004)
  arc A2974 (9.4636, 15.564) -> (9.441, 15.6367) centre (9.4523, 15.6004) ccw
  arc A2975 (8.8553, 15.4542) -> (8.8779, 15.3815) centre (8.8666, 15.4179) ccw
  line L1487 (9.4523, 15.6004) -> (10.0557, 15.711)
  arc A2976 (10.0625, 15.6735) -> (10.0488, 15.7484) centre (10.0557, 15.7109) ccw
  arc A2977 (9.4454, 15.6379) -> (9.4591, 15.5629) centre (9.4523, 15.6004) ccw
  line L1488 (10.0557, 15.711) -> (10.668, 15.748)
  arc A2978 (10.6703, 15.71) -> (10.6657, 15.786) centre (10.668, 15.748) ccw
  arc A2979 (10.0534, 15.749) -> (10.058, 15.6729) centre (10.0557, 15.711) ccw
  line L1489 (10.668, 15.748) -> (11.2803, 15.711)
  arc A2980 (11.278, 15.6729) -> (11.2826, 15.749) centre (11.2803, 15.711) ccw
  arc A2981 (10.6703, 15.786) -> (10.6657, 15.71) centre (10.668, 15.748) ccw
  line L1490 (11.2803, 15.711) -> (11.8837, 15.6004)
  arc A2982 (11.8769, 15.5629) -> (11.8906, 15.6379) centre (11.8837, 15.6004) ccw
  arc A2983 (11.2872, 15.7484) -> (11.2735, 15.6735) centre (11.2803, 15.7109) ccw
  line L1491 (11.8837, 15.6004) -> (12.4694, 15.4179)
  arc A2984 (12.4581, 15.3815) -> (12.4807, 15.4542) centre (12.4694, 15.4179) ccw
  arc A2985 (11.8951, 15.6367) -> (11.8724, 15.564) centre (11.8837, 15.6004) ccw
  line L1492 (12.4694, 15.4179) -> (13.0288, 15.1661)
  arc A2986 (13.0132, 15.1313) -> (13.0444, 15.2008) centre (13.0288, 15.1661) ccw
  arc A2987 (12.485, 15.4526) -> (12.4538, 15.3831) centre (12.4694, 15.4179) ccw
  line L1493 (13.0288, 15.1661) -> (13.5538, 14.8487)
  arc A2988 (13.5341, 14.8161) -> (13.5735, 14.8814) centre (13.5538, 14.8487) ccw
  arc A2989 (13.0485, 15.1987) -> (13.0091, 15.1335) centre (13.0288, 15.1661) ccw
  line L1494 (13.5538, 14.8487) -> (14.0367, 14.4704)
  arc A2990 (14.0132, 14.4404) -> (14.0602, 14.5004) centre (14.0367, 14.4704) ccw
  arc A2991 (13.5773, 14.8787) -> (13.5303, 14.8187) centre (13.5538, 14.8487) ccw
  line L1495 (14.0367, 14.4704) -> (14.4704, 14.0367)
  arc A2992 (14.4435, 14.0097) -> (14.4974, 14.0636) centre (14.4704, 14.0367) ccw
  arc A2993 (14.0636, 14.4974) -> (14.0097, 14.4435) centre (14.0367, 14.4704) ccw
  line L1496 (14.4704, 14.0367) -> (14.8488, 13.5538)
  arc A2994 (14.8188, 13.5303) -> (14.8788, 13.5773) centre (14.8488, 13.5538) ccw
  arc A2995 (14.5004, 14.0602) -> (14.4405, 14.0132) centre (14.4704, 14.0367) ccw
  line L1497 (14.8488, 13.5538) -> (15.1661, 13.0288)
  arc A2996 (15.1335, 13.0091) -> (15.1987, 13.0485) centre (15.1661, 13.0288) ccw
  arc A2997 (14.8814, 13.5735) -> (14.8162, 13.5341) centre (14.8488, 13.5538) ccw